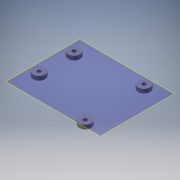
# Autodesk Inventor part: ChassisPrototypeA4
Saved by Autodesk Inventor 2017 (Build 210142000, 142)
## iProperties
Created: 2018-04-24
Part Number: ChassisPrototypeA4
Material: Generic
Document SubType Name: Modeling
Designer: MtgSaber
Density: 1 g/cm^3
Appearance: Default
Author: MtgSaber
Autodesk Inventor part; units mm, degrees
ref_plane "Work Plane1" through (50.6765, 0, 41.694) normal (0, -1, 0) x (-1, 0, 0)
ref_plane "Work Plane2" through (50.6765, -3.175, 41.694) normal (0, -1, 0) x (-1, 0, 0)
sketch "Sketch2" plane through (50.6765, -3.175, 41.694) normal (0, -1, 0) x (-1, 0, 0)
  circle A0 centre (32.579, -9.106) radius 1.5875 construction
  circle A1 centre (32.579, 18.834) radius 1.5875 construction
  circle A2 centre (-18.221, 23.914) radius 1.5875 construction
  circle A3 centre (-19.491, -24.346) radius 1.5875 construction
  line L0 (-33.461, 26.454) -> (-33.461, -26.886) construction
  line L1 (-33.461, -26.886) -> (30.039, -26.886) construction
  line L2 (30.039, -26.886) -> (32.579, -24.346) construction
  line L3 (32.579, -24.346) -> (32.579, -12.916) construction
  line L4 (32.579, -12.916) -> (35.119, -10.376) construction
  line L5 (35.119, -10.376) -> (35.119, 20.104) construction
  line L6 (35.119, 20.104) -> (32.579, 22.644) construction
  line L7 (32.579, 22.644) -> (32.579, 26.454) construction
  line L8 (32.579, 26.454) -> (-33.461, 26.454) construction
  circle A4 centre (32.579, -9.106) radius 1.5875
  circle A5 centre (-18.221, 23.914) radius 1.5875
  circle A6 centre (32.579, 18.834) radius 1.5875
  circle A7 centre (32.579, -9.106) radius 4.7625
  circle A8 centre (32.579, 18.834) radius 4.7625
  circle A9 centre (-18.221, 23.914) radius 4.7625
  circle A10 centre (-19.491, -24.346) radius 1.5875
  circle A11 centre (-19.491, -24.346) radius 4.7625
  point P0 (50.6765, 41.694)
  dimension "d7" = 9.525
  dimension "d8" = 9.525
  dimension "d9" = 9.525
  dimension "d10" = 3.175
  dimension "d11" = 9.525
  constraints: 18 end point, 12 centre point, 8 coincident, 4 concentric
  measures "d7" diameter of A7
  measures "d8" diameter of A8
  measures "d9" diameter of A9
  measures "d10" radial gap between concentric circles of A9 A5
  measures "d11" diameter of A11
extrude "Extrusion2" add sketch "Sketch2" along normal blind 3.175
ref_plane "Work Plane7" through (18.0975, -3.175, 36.83) normal (0, 0, 1) x (1, 0, 0)
ref_plane "Work Plane4" through (18.0975, -3.175, 27.6225) normal (0, 0, 1) x (1, 0, 0)
ref_plane "Work Plane6" through (18.0975, -3.175, 46.0375) normal (0, 0, -1) x (-1, 0, 0)
sketch "Sketch3" plane through (18.0975, -3.175, 36.83) normal (0, 0, 1) x (1, 0, 0)
  line L0 (46.0375, -3.175) -> (55.5625, -3.175) construction
  line L1 (55.5625, 0) -> (46.0375, 0) construction
  line L2 (-4.7625, -3.175) -> (4.7625, -3.175) construction
  line L3 (4.7625, 0) -> (-4.7625, 0) construction
  line L4 (46.0375, -3.175) -> (4.7625, -3.175) construction
  line L5 (4.7625, 0) -> (4.7625, -3.175) construction
  line L6 (25.4, -3.175) -> (25.4, -15.875) construction
  circle A0 centre (25.4, -9.525) radius 2.0574
  circle A1 centre (25.4, -9.525) radius 6.35 construction
  circle A2 centre (12.7, -9.525) radius 2.0574
  arc A3 (6.35, -9.525) -> (12.7, -15.875) centre (12.7, -9.525) ccw
  circle A4 centre (38.1, -9.525) radius 2.0574
  arc A5 (38.1, -15.875) -> (44.45, -9.525) centre (38.1, -9.525) ccw
  line L7 (38.1, -15.875) -> (12.7, -15.875)
  line L8 (44.45, -9.525) -> (44.45, -3.175)
  line L9 (6.35, -9.525) -> (6.35, -3.175)
  line L10 (44.45, -3.175) -> (6.35, -3.175)
  point P0 (-18.0975, 3.175)
  dimension "d14" = 4.1148
  dimension "d15" = 12.7
  dimension "d16" = 4.1148
  dimension "d17" = 12.7
  constraints: 12 end point, 7 tangent, 6 centre point, 4 point on circle, 3 coincident, 3 perpendicular, 2 midpoint, 2 point on line, 2 symmetric about line, 2 vertical, 2 other
  measures "d14" diameter of A0
  measures "d15" diameter of A1
  measures "d16" diameter of A2
  measures "d17" diameter of A3
extrude "Extrusion3" add sketch "Sketch3" along normal mid plane 4.7625
sketch "Sketch4" plane through (68.8975, -3.175, 17.78) normal (0, 1, 0) x (1, 0, 0)
  circle A0 centre (1.27, -48.26) radius 4.7625 construction
  circle A1 centre (1.27, -48.26) radius 1.5875 construction
  circle A2 centre (0, 0) radius 1.5875 construction
  circle A3 centre (0, 0) radius 4.7625 construction
  circle A4 centre (-50.8, -5.08) radius 1.5875 construction
  circle A5 centre (-50.8, -5.08) radius 4.7625 construction
  circle A6 centre (-50.8, -33.02) radius 4.7625 construction
  circle A7 centre (-50.8, -33.02) radius 1.5875 construction
  line L0 (-44.45, -16.6687) -> (-6.35, -16.6687) construction
  line L1 (-6.35, -21.4312) -> (-44.45, -21.4312) construction
  line L2 (-44.45, -21.4312) -> (-44.45, -16.6687) construction
  line L3 (-6.35, -21.4312) -> (-6.35, -16.6687) construction
  line L4 (-6.35, -19.05) -> (-44.45, -19.05) construction
  line L5 (-50.8, -33.02) -> (-33.3375, -19.05) construction
  line L6 (-33.3375, -19.05) -> (-50.8, -5.08) construction
  circle A8 centre (0, 0) radius 1.5875 construction
  line L7 (0, 0) -> (-17.4625, -19.05) construction
  circle A9 centre (1.27, -48.26) radius 1.5875 construction
  line L8 (1.27, -48.26) -> (-17.4625, -19.05) construction
  line L9 (-27.4574, -16.6687) -> (-23.3426, -16.6687) construction
  line L10 (-23.3426, -21.4312) -> (-27.4574, -21.4312) construction
  line L11 (-25.4, -21.4312) -> (-25.4, -16.6687) construction
  line L12 (-47.625, -13.4937) -> (-47.625, -24.6062)
  line L13 (-3.175, -24.6062) -> (-3.175, -13.4937)
  line L14 (-2.961, -46.0736) -> (-16.7281, -24.6062)
  line L15 (-15.5996, -13.4937) -> (-4.5423, -1.4313)
  line L16 (-9.1389, -13.4937) -> (-1.0316, -4.6494)
  line L17 (1.048, -43.5027) -> (-11.0704, -24.6062)
  arc A10 (1.048, -43.5027) -> (-2.961, -46.0736) centre (1.27, -48.26) ccw
  arc A11 (-4.5423, -1.4313) -> (-1.0316, -4.6494) centre (0, 0) ccw
  line L18 (-36.471, -24.6062) -> (-46.0918, -32.3029)
  circle A12 centre (-50.8, -33.02) radius 4.7625 construction
  line L19 (-49.0669, -28.584) -> (-44.0947, -24.6062)
  line L20 (-36.471, -13.4937) -> (-46.0918, -5.7971)
  line L21 (-44.0947, -13.4937) -> (-49.0669, -9.516)
  arc A13 (-46.0918, -32.3029) -> (-49.0669, -28.584) centre (-50.8, -33.02) ccw
  arc A14 (-49.0669, -9.516) -> (-46.0918, -5.7971) centre (-50.8, -5.08) ccw
  line L22 (-47.625, -24.6062) -> (-44.0947, -24.6062)
  line L23 (-44.0947, -13.4937) -> (-47.625, -13.4937)
  line L24 (-3.175, -13.4937) -> (-9.1389, -13.4937)
  line L25 (-15.5996, -13.4937) -> (-36.471, -13.4937)
  line L26 (-36.471, -24.6062) -> (-16.7281, -24.6062)
  line L27 (-11.0704, -24.6062) -> (-3.175, -24.6062)
  point P0 (-68.8975, 17.78)
  dimension "d20" = 15.875
  dimension "d21" = 7.9375
  dimension "d28" = 2.3813
  dimension "d29" = 2.3813
  dimension "d30" = 2.3813
  dimension "d31" = 2.3813
  dimension "d32" = 2.3813
  dimension "d33" = 2.3813
  dimension "d34" = 2.3813
  dimension "d35" = 2.3813
  dimension "d36" = 3.175
  dimension "d37" = 3.175
  dimension "d38" = 3.175
  dimension "d39" = 3.175
  constraints: 44 end point, 18 point on circle, 6 parallel, 4 centre point, 4 coincident, 4 collinear, 4 midpoint, 2 point on line
  measures "d20" distance of L7.end L5.end
  measures "d21" distance from line of L11 L5.end
  measures "d28" distance between parallel lines of L5 L18
  measures "d29" distance between parallel lines of L5 L19
  measures "d30" distance between parallel lines of L8 L17
  measures "d31" distance between parallel lines of L8 L14
  measures "d32" distance between parallel lines of L7 L15
  measures "d33" distance between parallel lines of L7 L16
  measures "d34" distance between parallel lines of L6 L20
  measures "d35" distance between parallel lines of L6 L21
  measures "d36" distance between parallel lines of L2 L12
  measures "d37" distance between parallel lines of L3 L13
  measures "d38" distance between parallel lines of L0 L25
  measures "d39" distance between parallel lines of L1 L26
extrude "Extrusion4" add sketch "Sketch4" against normal up to surface (3.175 mm away)
fillet "Fillet1" radius 1.5875 12 edges at (24.8028, -4.7625, 42.3862) (24.8028, -4.7625, 31.2737) (53.2979, -4.7625, 31.2737) (52.1694, -4.7625, 42.3862) (32.4265, -4.7625, 31.2737) (57.8271, -4.7625, 42.3862) (32.4265, -4.7625, 42.3862) (59.7586, -4.7625, 31.2737) (65.7225, -4.7625, 31.2737) (65.7225, -4.7625, 42.3862) (21.2725, -4.7625, 31.2737) (21.2725, -4.7625, 42.3862)
fillet "Fillet2" radius 1.5875 2 edges at (24.4475, -6.35, 36.83) (62.5475, -6.35, 36.83)
ref_plane "Work Plane3" through (20.6375, 0, 68.58) normal (0, 0, 1) x (1, 0, 0)
ref_plane "Work Plane5" through (84.1375, 0, 15.24) normal (0, 0, -1) x (-1, 0, 0)
body "Solid2"
